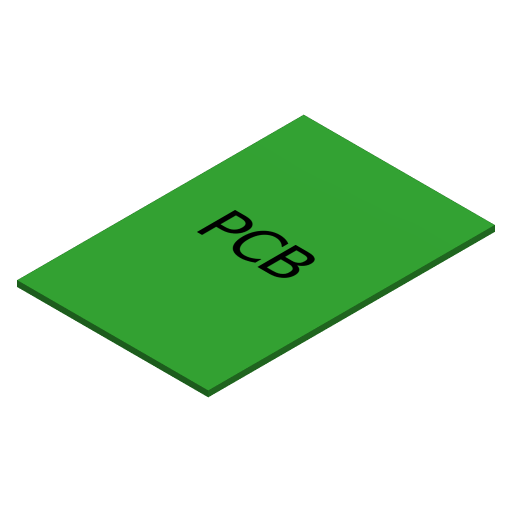
# Autodesk Inventor part: COTS_GENERIC_PCB
Saved by Autodesk Inventor 2024.3 (Build 283343000, 343)
## iProperties
Created: 2018-02-17
Part Number: COTS_GENERIC_PCB
Material: Ogólny
Document SubType Name: Modeling
Designer: Andrzej
Density: 1 g/cm^3
Appearance: Gładki - ciemna zieleń leśna
Author: Andrzej
Autodesk Inventor part; units mm, degrees
ref_plane "YZ Plane" through (0, 0, 0) normal (1, 0, 0) x (0, 1, 0)
ref_plane "XZ Plane" through (0, 0, 0) normal (0, 1, 0) x (-1, 0, 0)
ref_plane "XY Plane" through (0, 0, 0) normal (0, 0, 1) x (1, 0, 0)
sketch "Szkic1" plane through (0, 0, 0) normal (0, 0, 1) x (1, 0, 0)
  line L0 (-12.898, 5.4649) -> (37.102, 5.4649)
  line L1 (37.102, 5.4649) -> (37.102, -69.5351)
  line L2 (37.102, -69.5351) -> (-12.898, -69.5351)
  line L3 (-12.898, -69.5351) -> (-12.898, 5.4649)
  point P0 (0, 0)
  dimension "d0" = 50
  dimension "d1" = 75
  constraints: 8 end point, 2 parallel, 1 horizontal, 1 perpendicular
  measures "d0" distance of L1.end L2.end
  measures "d1" distance of L0.end L1.end
extrude "Wyciągnięcie proste1" add sketch "Szkic1" along normal blind 1.5
sketch "Szkic2" plane through (0, 0, 1.5) normal (0, 0, 1) x (1, 0, 0)
  line L0 (-1.3415, -24.8989) -> (31.392, -24.8989) construction
  line L1 (31.392, -24.8989) -> (31.392, -76.414) construction
  line L2 (31.392, -76.414) -> (-1.3415, -76.414) construction
  line L3 (-1.3415, -76.414) -> (-1.3415, -24.8989) construction
  constraints: 2 other
